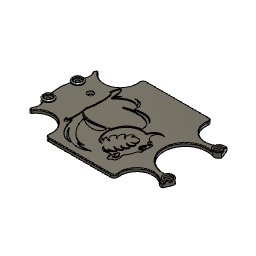
_chassis top.694dd02e-d549-4da8-af4c-a41191be3cab (Autodesk Fusion 360 design; units mm, degrees)
Autodesk Fusion 360 part; units mm, degrees
sketch "reference" plane through (0, 0, 0) normal (0, 1, 0) x (1, 0, 0)
  line L0 (26.708, 42.6236) -> (27.1586, 42.6236)
  line L1 (-27.225, -55.0823) -> (17.225, -55.0823)
  line L2 (17.225, -55.0823) -> (17.225, -42.3823)
  line L3 (17.225, -42.3823) -> (-27.225, -42.3823)
  line L4 (-27.225, -42.3823) -> (-27.225, -55.0823)
  circle A0 centre (0, 0) radius 65
  line L5 (-27.225, 55.0823) -> (17.225, 55.0823)
  line L6 (17.225, 55.0823) -> (17.225, 42.3823)
  line L7 (17.225, 42.3823) -> (-27.225, 42.3823)
  line L8 (-27.225, 55.0823) -> (-27.225, 42.3823)
  circle A1 centre (0, 0) radius 67.15
  circle A2 centre (68.0978, 18.2467) radius 3
  circle A3 centre (68.0978, 18.2467) radius 1.425
  line L9 (0, 0) -> (82, 0) construction
  line L10 (0, 0) -> (-41, 71.0141) construction
  line L11 (0, 0) -> (-41, -71.0141) construction
  line L12 (87.4769, -0.0257) -> (79.614, 0.0081)
  line L13 (-39.814, 68.9437) -> (-43.7162, 75.77)
  line L14 (-39.8, -68.9518) -> (-43.7607, -75.7444)
  line L15 (0, 0) -> (70.5, 0) construction
  arc A4 (79.614, 0.0081) -> (74.6944, -3.9877) centre (79.5926, -4.9919) ccw
  arc A5 (-39.814, 68.9437) -> (-33.8938, 66.6811) centre (-35.4732, 71.4251) ccw
  arc A6 (-39.8, -68.9518) -> (-40.8007, -62.6934) centre (-44.1194, -66.4332) ccw
  spline S0 degree 5 poles (-33.8938, 66.6811) (-33.483, 66.8179) (-33.0729, 66.9532) (-32.6634, 67.087) (-32.2547, 67.2193) (-31.8466, 67.3502) knots 0.021144 0.021144 0.021144 0.021144 0.021144 0.021144 0.032444 0.032444 0.032444 0.032444 0.032444 0.032444
  line L16 (-32.0549, 67.2834) -> (-31.6382, 67.417)
  spline S1 degree 5 poles (5.0849, 74.3263) (6.6179, 74.3731) (11.2429, 74.4207) (18.7539, 74.0099) (28.746, 72.2391) (40.5731, 67.6689) (52.3904, 59.5578) (62.916, 48.5693) (72.252, 34.9305) (78.8493, 22.0782) (83.3385, 11.4171) (86.1309, 3.8631) (87.4769, -0.0257) knots 0.251095 0.251095 0.251095 0.251095 0.251095 0.251095 0.3 0.4 0.5 0.6 0.7 0.8 0.9 1 1 1 1 1 1
  line L17 (-9.3123, 73.8863) -> (19.482, 74.7663)
  spline S2 degree 5 poles (-40.8007, -62.6934) (-41.1245, -62.4061) (-41.4467, -62.1186) (-41.7673, -61.8309) (-42.0863, -61.543) (-42.4037, -61.255) knots 0.021144 0.021144 0.021144 0.021144 0.021144 0.021144 0.032444 0.032444 0.032444 0.032444 0.032444 0.032444
  line L18 (-42.2416, -61.4021) -> (-42.5658, -61.1079)
  spline S3 degree 5 poles (-66.9109, -32.7595) (-67.718, -31.4553) (-70.0717, -27.4737) (-73.4714, -20.7636) (-76.9339, -11.2248) (-78.8895, 1.3029) (-77.7737, 15.5925) (-73.5202, 30.2022) (-66.3767, 45.1068) (-58.5449, 57.2464) (-51.5568, 66.4647) (-46.4109, 72.66) (-43.7162, 75.77) knots 0.251095 0.251095 0.251095 0.251095 0.251095 0.251095 0.3 0.4 0.5 0.6 0.7 0.8 0.9 1 1 1 1 1 1
  line L19 (-59.9171, -44.0611) -> (-73.9047, -21.4578)
  arc A7 (-66.9109, -32.7595) -> (-37.25, -64.5189) centre (0, 0) ccw
  spline S4 degree 5 poles (74.6944, -3.9877) (74.6075, -4.4118) (74.5196, -4.8346) (74.4308, -5.2561) (74.341, -5.6763) (74.2503, -6.0951) knots 0.021144 0.021144 0.021144 0.021144 0.021144 0.021144 0.032444 0.032444 0.032444 0.032444 0.032444 0.032444
  line L20 (74.2965, -5.8814) -> (74.204, -6.3089)
  spline S5 degree 5 poles (61.826, -41.5668) (61.1001, -42.9178) (58.8287, -46.947) (54.7175, -53.2463) (48.1879, -61.0143) (38.3164, -68.9717) (25.3834, -75.1503) (10.6042, -78.7715) (-5.8753, -80.0373) (-20.3044, -79.3246) (-31.7817, -77.8819) (-39.7199, -76.523) (-43.7607, -75.7444) knots 0.251095 0.251095 0.251095 0.251095 0.251095 0.251095 0.3 0.4 0.5 0.6 0.7 0.8 0.9 1 1 1 1 1 1
  line L21 (68.2252, -29.657) -> (55.4268, -53.4766)
  arc A8 (61.826, -41.5668) -> (74.5, 0) centre (0, 0) ccw
  arc A9 (5.0849, 74.3263) -> (-37.25, 64.5189) centre (0, 0) ccw
  circle A10 centre (18.2467, 68.0978) radius 3
  circle A11 centre (18.2467, 68.0978) radius 1.425
  circle A12 centre (-49.851, 49.851) radius 3
  circle A13 centre (-49.851, 49.851) radius 1.425
  circle A14 centre (-68.0978, -18.2467) radius 3
  circle A15 centre (-68.0978, -18.2467) radius 1.425
  circle A16 centre (-18.2467, -68.0978) radius 3
  circle A17 centre (-18.2467, -68.0978) radius 1.425
  circle A18 centre (49.851, -49.851) radius 3
  circle A19 centre (49.851, -49.851) radius 1.425
  line L22 (0, 0) -> (55.15, 0) construction
  line L23 (0, 0) -> (55.15, 0) construction
  circle A20 centre (42.2474, -35.4497) radius 12
  circle A21 centre (42.2474, 35.4497) radius 12
  line L24 (0, 0) -> (55.15, 0) construction
  line L25 (0, 0) -> (55.15, 0) construction
  circle A22 centre (-42.2474, 35.4497) radius 12
  circle A23 centre (-42.2474, -35.4497) radius 12
  circle A24 centre (0, 0) radius 62.5
  line L26 (-5, -42.3823) -> (-5, 42.3823)
  point P0 (39, 67.55)
  point P1 (-78, 0)
  point P2 (39, -67.55)
  dimension "d9" = 12.7
  dimension "d10" = 44.45
  dimension "d53" = 12.7
  dimension "d54" = 44.45
  dimension "d63" = 130
  dimension "d76" = 134.3
  dimension "d123" = 78
  dimension "d127" = 5
  dimension "d128" = 5
  dimension "d129" = 5
  dimension "d132" = 149
  dimension "d136" = 360
  dimension "d204" = 55.15
  dimension "d206" = 55.15
  dimension "d207" = 24
  dimension "d208" = 24
  dimension "d210" = 55.15
  dimension "d212" = 55.15
  dimension "d213" = 24
  dimension "d214" = 24
  dimension "d227" = 125
  dimension "d232" = 84.7646
  constraint perpendicular L1 L2
  constraint perpendicular L2 L3
  constraint coincident A0.centre A1.centre
  constraint perpendicular L5 L6
  constraint perpendicular L6 L7
  constraint horizontal L9
  constraint horizontal L15
  constraint tangent A4 S4
  constraint tangent L12 A4
  constraint tangent A5 S0
  constraint tangent L13 A5
  constraint tangent A6 S2
  constraint tangent L14 A6
  constraint coincident S0.end A7
  constraint midpoint S0.end L16
  constraint coincident S1.start A7
  constraint midpoint S1.start L17
  constraint coincident L10 A9.end
  constraint coincident S2.end A7
  constraint midpoint S2.end L18
  constraint midpoint S3.start L19
  constraint coincident L11 A7.end
  constraint concentric A7 A8
  constraint coincident S4.end A8
  constraint midpoint S4.end L20
  constraint midpoint S5.start L21
  constraint coincident L9 A8.end
  constraint concentric A8 A9
  constraint horizontal L22
  constraint horizontal L23
  constraint horizontal L24
  constraint horizontal L25
  constraint midpoint L3 L26.start
  constraint midpoint L7 L26.end
  constraint perpendicular L7 L26
  measures "d9" distance of L1.end L2.end
  measures "d10" distance of L2.end L3.end
  measures "d53" distance of L5.end L6.end
  measures "d54" distance of L6.end L7.end
  measures "d63" diameter of A0
  measures "d76" diameter of A1
  measures "d123" distance of A0.centre P0
  measures "d127" radius of A4
  measures "d128" radius of A5
  measures "d129" radius of A6
  measures "d132" diameter of A7
  measures "d204" distance of A0.centre A20.centre
  measures "d206" distance of A0.centre A21.centre
  measures "d207" diameter of A20
  measures "d208" diameter of A21
  measures "d210" distance of A0.centre A23.centre
  measures "d212" distance of A0.centre A22.centre
  measures "d213" diameter of A22
  measures "d214" diameter of A23
  measures "d227" diameter of A24
  measures "d232" distance of L26.start L26.end
sketch "Sketch6" plane through (0, 0, 0) normal (0, 1, 0) x (1, 0, 0)
  line L0 (25.9471, -41.0033) -> (-25.9305, -41.0033)
  arc A0 (53.3928, 17.0259) -> (53.3489, -17.1529) centre (47.6253, -0.0562) ccw
  arc A1 (-28.8946, -37.5404) -> (-53.2717, -27.6825) centre (-42.2338, -35.4569) ccw
  arc A2 (52.1423, -26.2602) -> (28.9106, -37.5367) centre (42.2443, -35.4374) ccw
  arc A3 (55.1761, 27.1684) -> (52.1143, 26.331) centre (54.3168, 24.2941) ccw
  arc A4 (52.1423, -26.2602) -> (55.2056, -27.0935) centre (54.3422, -24.2205) ccw
  arc A5 (58.3345, -19.4651) -> (53.3489, -17.1529) centre (54.6188, -20.946) ccw
  arc A6 (53.3928, 17.0259) -> (58.3852, 19.3275) centre (54.6724, 20.8157) ccw
  circle A7 centre (54.6724, 20.8157) radius 1.425
  circle A8 centre (54.6188, -20.946) radius 1.425
  arc A9 (-56.1762, -2.0025) -> (-56.1762, -2.0026) centre (-0.0106, -0.0004) ccw
  circle A10 centre (-54.8812, 12.3936) radius 1.425
  circle A11 centre (-54.8757, -12.1807) radius 1.425
  arc A12 (28.9662, 37.5373) -> (52.1143, 26.331) centre (42.246, 35.4576) ccw
  line L1 (-54.6751, -2.0026) -> (-54.4366, -2.0026) construction
  line L2 (-49.9389, 12.059) -> (-49.9913, 12.0592)
  line L3 (-44.9427, 8.8286) -> (-44.9427, 8.8286)
  spline S0 degree 5 poles (-38.2674, -23.601) (-38.2616, -23.5615) (-38.25, -23.4822) (-38.2328, -23.3629) (-38.21, -23.2029) (-38.1818, -23.0019) (-38.1594, -22.8402) (-38.1427, -22.7184) (-38.1316, -22.6368) (-38.1261, -22.596) knots 0 0 0 0 0 0 0.2 0.4 0.6 0.8 1 1 1 1 1 1
  line L4 (-38.2822, -23.7022) -> (-38.2526, -23.4999)
  line L5 (-38.1402, -22.7004) -> (-38.112, -22.4916)
  arc A13 (-53.2884, 27.6676) -> (-28.8973, 37.5386) centre (-42.2488, 35.4595) ccw
  line L6 (-54.333, 19.0252) -> (-54.7513, 17.7702)
  arc A14 (-56.8345, 14.6706) -> (-57.7304, 11.4541) centre (-54.8812, 12.3936) ccw
  spline S1 degree 3 poles (-57.5488, 7.7264) (-57.7948, 6.6323) (-57.9976, 5.5893) (-58.1533, 4.5869) (-58.73, 0.873) (-58.6151, -2.3643) (-57.8493, -6.2568) (-57.7624, -6.6981) (-57.6677, -7.149) (-57.5653, -7.6097) knots 0.254144 0.254144 0.254144 0.254144 0.280571 0.280571 0.280571 0.378481 0.378481 0.378481 0.389582 0.389582 0.389582 0.389582
  arc A15 (-57.7325, -11.2651) -> (-56.8532, -14.4367) centre (-54.8757, -12.1807) ccw
  spline S2 degree 3 poles (-54.8028, -17.5596) (-54.6442, -18.0533) (-54.4816, -18.5512) (-54.3154, -19.0517) knots 0.459488 0.459488 0.459488 0.459488 0.468931 0.468931 0.468931 0.468931
  arc A16 (-55.114, 16.8875) -> (-54.7513, 17.7702) centre (-61.3921, 19.9836) ccw
  arc A17 (-54.333, 19.0252) -> (-55.3983, 25.4709) centre (-60.9739, 21.2385) ccw
  arc A18 (-57.5488, 7.7264) -> (-57.4036, 8.667) centre (-64.3783, 9.2621) ccw
  arc A19 (-57.4291, -8.4753) -> (-57.5653, -7.6097) centre (-64.3985, -9.1286) ccw
  arc A20 (-54.8028, -17.5596) -> (-55.1565, -16.672) centre (-61.4673, -19.7007) ccw
  arc A21 (-55.3823, -25.4886) -> (-54.3154, -19.0517) centre (-60.9588, -21.2575) ccw
  arc A22 (-51.9311, -12.9587) -> (-51.9223, -12.9246) centre (-54.8757, -12.1807) ccw
  line L7 (-53.5111, 9.0025) -> (-53.3775, 9.0028)
  arc A23 (-53.5111, 9.0025) -> (-54.0242, 8.7111) centre (-53.5096, 8.4025) ccw
  line L8 (-25.9331, 41.0003) -> (26.0023, 41.0015)
  arc A24 (-55.4878, -26.5244) -> (-54.9832, -27.5548) centre (-0.0035, 0.0074) ccw
  arc A25 (-54.9996, 27.5386) -> (-55.5043, 26.5064) centre (-0.0035, 0.0074) ccw
  arc A26 (-53.2884, 27.6676) -> (-54.9996, 27.5386) centre (-54.1054, 27.0909) ccw
  arc A27 (-55.5043, 26.5064) -> (-55.3983, 25.4709) centre (-54.6018, 26.0756) ccw
  arc A28 (-54.9832, -27.5548) -> (-53.2717, -27.6825) centre (-54.0893, -27.1066) ccw
  arc A29 (-55.3823, -25.4886) -> (-55.4878, -26.5244) centre (-54.5856, -26.093) ccw
  arc A30 (55.2056, -27.0935) -> (58.3345, -19.4651) centre (-0.0035, 0.0074) ccw
  arc A31 (58.3852, 19.3275) -> (55.1761, 27.1684) centre (-0.0035, 0.0074) ccw
  arc A32 (-28.8946, -37.5404) -> (-25.9305, -41.0033) centre (-25.9305, -38.0033) ccw
  arc A33 (25.9471, -41.0033) -> (28.9106, -37.5367) centre (25.9471, -38.0033) ccw
  arc A34 (28.9662, 37.5373) -> (26.0023, 41.0015) centre (26.0024, 38.0015) ccw
  arc A35 (-25.9331, 41.0003) -> (-28.8973, 37.5386) centre (-25.9331, 38.0003) ccw
  circle A36 centre (-54.8812, 12.3936) radius 3
  circle A37 centre (-54.8757, -12.1807) radius 3
  circle A38 centre (-54.8812, 12.3936) radius 4.5
  circle A39 centre (-54.8757, -12.1807) radius 4.5
  arc A40 (51.5521, -17.6527) -> (56.0971, -25.1962) centre (54.6188, -20.946) ccw
  arc A41 (56.1643, 25.0612) -> (51.5973, 17.5303) centre (54.6724, 20.8157) ccw
  arc A42 (57.2747, 22.4063) -> (57.6738, 21.3577) centre (54.6724, 20.8157) ccw
  arc A43 (57.6206, -21.4861) -> (57.2117, -22.552) centre (54.6188, -20.946) ccw
  circle A44 centre (-40.8812, 8.8936) radius 2.5
  spline S3 degree 3 poles (23.3331, -3.4893) (23.2569, -3.2607) (23.0664, -2.9273) (22.895, -2.7559) knots 0 0 0 0 1 1 1 1
  spline S4 degree 3 poles (22.895, -2.7559) (22.1997, -2.0415) (21.2948, -2.2891) (20.3042, -3.4798) knots 0 0 0 0 1 1 1 1
  line L9 (20.3042, -3.4798) -> (20.0375, -3.7941)
  line L10 (20.0375, -3.7941) -> (19.7803, -3.556)
  spline S5 degree 3 poles (19.7803, -3.556) (19.6374, -3.4321) (19.4088, -3.2512) (19.2755, -3.1654) knots 0 0 0 0 1 1 1 1
  spline S6 degree 3 poles (19.2755, -3.1654) (19.0374, -3.0226) (18.5516, -2.3653) (18.6278, -2.2987) knots 0 0 0 0 1 1 1 1
  spline S7 degree 3 poles (18.6278, -2.2987) (18.6468, -2.2891) (18.8564, -2.1748) (19.0945, -2.0605) knots 0 0 0 0 1 1 1 1
  spline S8 degree 3 poles (19.0945, -2.0605) (19.5708, -1.8224) (20.7138, -1.0795) (20.7138, -1.0033) knots 0 0 0 0 1 1 1 1
  spline S9 degree 3 poles (20.7138, -1.0033) (20.7138, -0.9747) (20.5137, -0.9652) (20.2661, -0.9842) knots 0 0 0 0 1 1 1 1
  spline S10 degree 3 poles (20.2661, -0.9842) (19.647, -1.0318) (18.6087, -0.7747) (17.942, -0.4222) knots 0 0 0 0 1 1 1 1
  spline S11 degree 3 poles (17.942, -0.4222) (16.9228, 0.1302) (16.0179, 1.2923) (15.7036, 2.4734) knots 0 0 0 0 1 1 1 1
  spline S12 degree 3 poles (15.7036, 2.4734) (15.5322, 3.1115) (15.5417, 4.1593) (15.7131, 4.8546) knots 0 0 0 0 1 1 1 1
  spline S13 degree 3 poles (15.7131, 4.8546) (16.1703, 6.6072) (17.6753, 8.0074) (19.5136, 8.3979) knots 0 0 0 0 1 1 1 1
  spline S14 degree 3 poles (19.5136, 8.3979) (19.9137, 8.4836) (20.3994, 8.5122) (20.7138, 8.4836) knots 0 0 0 0 1 1 1 1
  line L11 (20.7138, 8.4836) -> (21.2376, 8.4265)
  line L12 (21.2376, 8.4265) -> (20.8852, 8.617)
  spline S15 degree 3 poles (20.8852, 8.617) (19.7803, 9.2075) (17.9134, 9.2552) (16.5609, 8.7218) knots 0 0 0 0 1 1 1 1
  spline S16 degree 3 poles (16.5609, 8.7218) (14.694, 7.9979) (13.2747, 6.6644) (12.3889, 4.8165) knots 0 0 0 0 1 1 1 1
  spline S17 degree 3 poles (12.3889, 4.8165) (12.2079, 4.426) (12.0079, 3.8926) (11.9412, 3.6164) knots 0 0 0 0 1 1 1 1
  line L13 (11.9412, 3.6164) -> (11.8269, 3.1115)
  line L14 (11.8269, 3.1115) -> (11.2935, 3.2925)
  spline S18 degree 3 poles (11.2935, 3.2925) (9.579, 3.8831) (6.9692, 4.0736) (5.1309, 3.7307) knots 0 0 0 0 1 1 1 1
  spline S19 degree 3 poles (5.1309, 3.7307) (-2.8225, 2.2638) (-8.0613, -6.3468) (-6.2229, -14.9098) knots 0 0 0 0 1 1 1 1
  spline S20 degree 3 poles (-6.2229, -14.9098) (-5.8801, -16.5195) (-5.1943, -18.3673) (-4.2322, -20.32) knots 0 0 0 0 1 1 1 1
  spline S21 degree 3 poles (-4.2322, -20.32) (-3.6226, -21.5392) (-2.4034, -22.4345) (-1.2318, -22.5107) knots 0 0 0 0 1 1 1 1
  spline S22 degree 3 poles (-1.2318, -22.5107) (-0.6318, -22.5488) (-0.0508, -22.425) (0.1207, -22.2154) knots 0 0 0 0 1 1 1 1
  spline S23 degree 3 poles (0.1207, -22.2154) (0.1969, -22.1297) (0.1112, -22.1011) (-0.1841, -22.0916) knots 0 0 0 0 1 1 1 1
  spline S24 degree 3 poles (-0.1841, -22.0916) (-1.6891, -22.0535) (-3.1845, -20.4724) (-3.4131, -18.7007) knots 0 0 0 0 1 1 1 1
  spline S25 degree 3 poles (-3.4131, -18.7007) (-3.4512, -18.4245) (-3.4416, -18.2435) (-3.3845, -18.2435) knots 0 0 0 0 1 1 1 1
  spline S26 degree 3 poles (-3.3845, -18.2435) (-3.3274, -18.2435) (-3.2893, -18.3007) (-3.2893, -18.3769) knots 0 0 0 0 1 1 1 1
  spline S27 degree 3 poles (-3.2893, -18.3769) (-3.2893, -18.4531) (-3.0702, -18.7483) (-2.813, -19.0436) knots 0 0 0 0 1 1 1 1
  spline S28 degree 3 poles (-2.813, -19.0436) (-2.3368, -19.558) (-1.9176, -19.7866) (-1.2128, -19.9009) knots 0 0 0 0 1 1 1 1
  spline S29 degree 3 poles (-1.2128, -19.9009) (-0.8889, -19.958) (-0.7842, -19.8151) (-1.089, -19.7199) knots 0 0 0 0 1 1 1 1
  spline S30 degree 3 poles (-1.089, -19.7199) (-1.3747, -19.6342) (-2.0415, -18.8531) (-2.2415, -18.3864) knots 0 0 0 0 1 1 1 1
  spline S31 degree 3 poles (-2.2415, -18.3864) (-2.5082, -17.7768) (-2.6416, -16.8719) (-2.5653, -16.2814) knots 0 0 0 0 1 1 1 1
  line L15 (-2.5654, -16.2814) -> (-2.5082, -15.7575)
  line L16 (-2.5082, -15.7575) -> (-2.1843, -16.1385)
  spline S32 degree 3 poles (-2.1843, -16.1385) (-1.4033, -17.0529) (-0.0222, -17.672) (1.2256, -17.672) knots 0 0 0 0 1 1 1 1
  spline S33 degree 3 poles (1.2256, -17.672) (2.0162, -17.672) (2.3496, -17.5387) (1.7876, -17.4529) knots 0 0 0 0 1 1 1 1
  spline S34 degree 3 poles (1.7876, -17.4529) (0.8256, -17.3005) (-0.4984, -16.2718) (-0.9937, -15.3098) knots 0 0 0 0 1 1 1 1
  spline S35 degree 3 poles (-0.9937, -15.3098) (-1.8986, -13.5477) (-1.4033, -11.6427) (0.1588, -10.8712) knots 0 0 0 0 1 1 1 1
  line L17 (0.1588, -10.8712) -> (0.6446, -10.6235)
  line L18 (0.6446, -10.6235) -> (0.9494, -11.0807)
  spline S36 degree 3 poles (0.9494, -11.0807) (1.359, -11.6808) (2.0162, -12.2713) (2.6067, -12.5666) knots 0 0 0 0 1 1 1 1
  spline S37 degree 3 poles (2.6067, -12.5666) (2.8734, -12.7) (3.1116, -12.8143) (3.1497, -12.8143) knots 0 0 0 0 1 1 1 1
  spline S38 degree 3 poles (3.1497, -12.8143) (3.1878, -12.8143) (3.0163, -12.6047) (2.7782, -12.3475) knots 0 0 0 0 1 1 1 1
  spline S39 degree 3 poles (2.7782, -12.3475) (1.178, -10.6426) (1.3209, -7.8898) (3.083, -6.5563) knots 0 0 0 0 1 1 1 1
  spline S40 degree 3 poles (3.083, -6.5563) (3.3021, -6.3849) (3.5402, -6.242) (3.6164, -6.242) knots 0 0 0 0 1 1 1 1
  spline S41 degree 3 poles (3.6164, -6.242) (3.6831, -6.242) (3.7878, -6.442) (3.845, -6.6802) knots 0 0 0 0 1 1 1 1
  spline S42 degree 3 poles (3.845, -6.6802) (4.1879, -8.0422) (5.4357, -9.3472) (6.6644, -9.6329) knots 0 0 0 0 1 1 1 1
  spline S43 degree 3 poles (6.6644, -9.6329) (6.9501, -9.6996) (6.9501, -9.6901) (6.5501, -9.3472) knots 0 0 0 0 1 1 1 1
  spline S44 degree 3 poles (6.5501, -9.3472) (5.3118, -8.2708) (4.8546, -6.3849) (5.4928, -4.9942) knots 0 0 0 0 1 1 1 1
  spline S45 degree 3 poles (5.4928, -4.9942) (6.0072, -3.8798) (6.7501, -3.3845) (7.9122, -3.3845) knots 0 0 0 0 1 1 1 1
  spline S46 degree 3 poles (7.9122, -3.3845) (8.2932, -3.3845) (8.6361, -3.4321) (8.6646, -3.4798) knots 0 0 0 0 1 1 1 1
  spline S47 degree 3 poles (8.6646, -3.4798) (8.6932, -3.5369) (8.6361, -3.7084) (8.5218, -3.8608) knots 0 0 0 0 1 1 1 1
  spline S48 degree 3 poles (8.5218, -3.8608) (8.2646, -4.2227) (7.9503, -5.1085) (7.9503, -5.4514) knots 0 0 0 0 1 1 1 1
  spline S49 degree 3 poles (7.9503, -5.4514) (7.9598, -5.7181) (7.9598, -5.7181) (8.1408, -5.3752) knots 0 0 0 0 1 1 1 1
  spline S50 degree 3 poles (8.1408, -5.3752) (8.5408, -4.6228) (9.5695, -3.956) (10.6649, -3.756) knots 0 0 0 0 1 1 1 1
  spline S51 degree 3 poles (10.6649, -3.756) (11.7126, -3.5655) (12.989, -3.9465) (13.7224, -4.6799) knots 0 0 0 0 1 1 1 1
  spline S52 degree 3 poles (13.7224, -4.6799) (15.2369, -6.2039) (14.4939, -8.6423) (12.2841, -9.3853) knots 0 0 0 0 1 1 1 1
  line L19 (12.2841, -9.3853) -> (11.7126, -9.5758)
  line L20 (11.7126, -9.5758) -> (12.4746, -9.5472)
  spline S53 degree 3 poles (12.4746, -9.5472) (13.2938, -9.4996) (14.0653, -9.2614) (14.6749, -8.8519) knots 0 0 0 0 1 1 1 1
  spline S54 degree 3 poles (14.6749, -8.8519) (15.0845, -8.5756) (15.1321, -8.6137) (15.275, -9.29) knots 0 0 0 0 1 1 1 1
  spline S55 degree 3 poles (15.275, -9.29) (15.456, -10.1187) (15.0369, -11.1474) (14.3034, -11.6808) knots 0 0 0 0 1 1 1 1
  spline S56 degree 3 poles (14.3034, -11.6808) (13.1985, -12.4809) (11.7984, -12.6142) (10.5982, -12.0142) knots 0 0 0 0 1 1 1 1
  spline S57 degree 3 poles (10.5982, -12.0142) (10.341, -11.8999) (10.141, -11.8237) (10.141, -11.8713) knots 0 0 0 0 1 1 1 1
  spline S58 degree 3 poles (10.141, -11.8713) (10.141, -12.0618) (11.2459, -12.919) (11.7412, -13.1095) knots 0 0 0 0 1 1 1 1
  spline S59 degree 3 poles (11.7412, -13.1095) (12.3794, -13.3477) (13.4462, -13.4429) (14.0463, -13.3) knots 0 0 0 0 1 1 1 1
  spline S60 degree 3 poles (14.0463, -13.3) (14.2749, -13.2524) (14.4844, -13.2238) (14.5035, -13.2334) knots 0 0 0 0 1 1 1 1
  spline S61 degree 3 poles (14.5035, -13.2334) (14.6273, -13.3572) (14.6178, -14.0239) (14.4749, -14.4811) knots 0 0 0 0 1 1 1 1
  spline S62 degree 3 poles (14.4749, -14.4811) (13.9796, -16.1956) (11.5126, -17.0529) (9.7886, -16.1004) knots 0 0 0 0 1 1 1 1
  spline S63 degree 3 poles (9.7886, -16.1004) (9.56, -15.9766) (9.379, -15.9099) (9.379, -15.948) knots 0 0 0 0 1 1 1 1
  spline S64 degree 3 poles (9.379, -15.948) (9.379, -16.129) (10.3791, -16.9386) (10.884, -17.1767) knots 0 0 0 0 1 1 1 1
  spline S65 degree 3 poles (10.884, -17.1767) (11.3697, -17.4053) (11.5412, -17.4339) (12.4461, -17.4339) knots 0 0 0 0 1 1 1 1
  spline S66 degree 3 poles (12.4461, -17.4339) (13.2081, -17.4339) (13.4748, -17.4625) (13.4748, -17.5577) knots 0 0 0 0 1 1 1 1
  spline S67 degree 3 poles (13.4748, -17.5577) (13.4748, -17.8339) (13.0176, -18.615) (12.608, -19.0246) knots 0 0 0 0 1 1 1 1
  spline S68 degree 3 poles (12.608, -19.0246) (11.4078, -20.2247) (9.4742, -20.4914) (7.8264, -19.6723) knots 0 0 0 0 1 1 1 1
  line L21 (7.8264, -19.6723) -> (7.2835, -19.396)
  line L22 (7.2835, -19.396) -> (7.474, -19.6723)
  spline S69 degree 3 poles (7.474, -19.6723) (8.1693, -20.6438) (9.56, -21.3201) (10.9221, -21.3296) knots 0 0 0 0 1 1 1 1
  spline S70 degree 3 poles (10.9221, -21.3296) (11.3316, -21.3391) (11.665, -21.3487) (11.665, -21.3677) knots 0 0 0 0 1 1 1 1
  spline S71 degree 3 poles (11.665, -21.3677) (11.665, -21.5392) (11.1602, -22.2821) (10.7697, -22.6726) knots 0 0 0 0 1 1 1 1
  spline S72 degree 3 poles (10.7697, -22.6726) (9.8743, -23.5775) (8.5884, -23.9966) (7.2359, -23.8537) knots 0 0 0 0 1 1 1 1
  spline S73 degree 3 poles (7.2359, -23.8537) (6.9216, -23.8156) (6.6549, -23.7966) (6.6358, -23.8156) knots 0 0 0 0 1 1 1 1
  spline S74 degree 3 poles (6.6358, -23.8156) (6.531, -23.9204) (8.0836, -24.5491) (8.5503, -24.5967) knots 0 0 0 0 1 1 1 1
  spline S75 degree 3 poles (8.5503, -24.5967) (9.0837, -24.6538) (9.0932, -24.6538) (8.9313, -24.8348) knots 0 0 0 0 1 1 1 1
  spline S76 degree 3 poles (8.9313, -24.8348) (8.8456, -24.9301) (8.5027, -25.1491) (8.1693, -25.3111) knots 0 0 0 0 1 1 1 1
  spline S77 degree 3 poles (8.1693, -25.3111) (6.5977, -26.0826) (4.5403, -25.6063) (3.2925, -24.1871) knots 0 0 0 0 1 1 1 1
  spline S78 degree 3 poles (3.2925, -24.1871) (2.8258, -23.6537) (2.8258, -23.7871) (3.283, -24.7681) knots 0 0 0 0 1 1 1 1
  spline S79 degree 3 poles (3.283, -24.7681) (3.7878, -25.8635) (4.826, -26.7398) (6.0643, -27.1113) knots 0 0 0 0 1 1 1 1
  spline S80 degree 3 poles (6.0643, -27.1113) (7.0644, -27.4161) (8.3312, -27.3494) (9.2361, -26.9303) knots 0 0 0 0 1 1 1 1
  spline S81 degree 3 poles (9.2361, -26.9303) (9.6076, -26.7589) (10.2267, -26.5398) (10.6173, -26.435) knots 0 0 0 0 1 1 1 1
  spline S82 degree 3 poles (10.6173, -26.435) (11.0078, -26.3398) (11.4174, -26.2255) (11.5221, -26.1969) knots 0 0 0 0 1 1 1 1
  spline S83 degree 3 poles (11.5221, -26.1969) (11.7031, -26.1397) (11.7126, -26.1969) (11.7412, -26.9779) knots 0 0 0 0 1 1 1 1
  spline S84 degree 3 poles (11.7412, -26.9779) (11.8174, -28.921) (12.4461, -30.5784) (13.3128, -31.1023) knots 0 0 0 0 1 1 1 1
  spline S85 degree 3 poles (13.3128, -31.1023) (13.6748, -31.3309) (14.3225, -31.3499) (14.7035, -31.1499) knots 0 0 0 0 1 1 1 1
  spline S86 degree 3 poles (14.7035, -31.1499) (15.0464, -30.9784) (15.6083, -30.3212) (15.837, -29.8545) knots 0 0 0 0 1 1 1 1
  spline S87 degree 3 poles (15.837, -29.8545) (15.9989, -29.5021) (15.9989, -29.5021) (16.4847, -29.5497) knots 0 0 0 0 1 1 1 1
  spline S88 degree 3 poles (16.4847, -29.5497) (17.3229, -29.6354) (17.761, -29.2544) (18.0849, -28.159) knots 0 0 0 0 1 1 1 1
  spline S89 degree 3 poles (18.0849, -28.159) (18.4659, -26.8636) (18.3325, -25.0729) (17.7134, -23.2251) knots 0 0 0 0 1 1 1 1
  line L23 (17.7134, -23.2251) -> (17.38, -22.225)
  line L24 (17.38, -22.225) -> (17.7515, -21.7773)
  spline S90 degree 3 poles (17.7515, -21.7773) (18.8183, -20.5009) (19.8946, -18.5293) (20.4661, -16.8148) knots 0 0 0 0 1 1 1 1
  spline S91 degree 3 poles (20.4661, -16.8148) (20.7995, -15.8146) (21.19, -14.1001) (21.19, -13.6334) knots 0 0 0 0 1 1 1 1
  spline S92 degree 3 poles (21.19, -13.6334) (21.19, -13.3953) (21.2186, -13.3858) (21.6663, -13.3858) knots 0 0 0 0 1 1 1 1
  spline S93 degree 3 poles (21.6663, -13.3858) (22.3235, -13.3858) (22.6473, -13.1953) (22.914, -12.6523) knots 0 0 0 0 1 1 1 1
  spline S94 degree 3 poles (22.914, -12.6523) (23.1141, -12.2428) (23.1426, -12.0713) (23.1426, -11.0045) knots 0 0 0 0 1 1 1 1
  spline S95 degree 3 poles (23.1426, -11.0045) (23.1331, -10.0996) (23.0855, -9.6329) (22.9331, -9.0614) knots 0 0 0 0 1 1 1 1
  spline S96 degree 3 poles (22.9331, -9.0614) (22.7426, -8.3661) (22.7331, -8.2804) (22.8664, -8.0232) knots 0 0 0 0 1 1 1 1
  spline S97 degree 3 poles (22.8664, -8.0232) (22.9521, -7.8708) (23.1236, -7.3374) (23.2474, -6.8421) knots 0 0 0 0 1 1 1 1
  spline S98 degree 3 poles (23.2474, -6.8421) (23.5141, -5.7943) (23.5522, -4.1941) (23.3331, -3.4893) knots 0 0 0 0 1 1 1 1
  spline S99 degree 3 poles (23.0474, -6.9564) (22.7045, -8.2994) (21.6567, -9.8139) (20.6661, -10.3949) knots 0 0 0 0 1 1 1 1
  spline S100 degree 3 poles (20.6661, -10.3949) (20.1804, -10.6807) (19.5136, -10.7759) (19.1898, -10.6045) knots 0 0 0 0 1 1 1 1
  spline S101 degree 3 poles (19.1898, -10.6045) (18.5706, -10.2711) (18.3325, -9.4329) (18.5611, -8.328) knots 0 0 0 0 1 1 1 1
  spline S102 degree 3 poles (18.5611, -8.328) (18.9326, -6.5754) (20.3232, -4.7656) (21.5901, -4.4323) knots 0 0 0 0 1 1 1 1
  spline S103 degree 3 poles (21.5901, -4.4323) (22.8188, -4.0989) (23.4855, -5.2514) (23.0474, -6.9564) knots 0 0 0 0 1 1 1 1
  spline S104 degree 3 poles (15.8846, -26.2636) (15.6369, -26.6827) (15.1512, -26.7398) (14.7416, -26.3969) knots 0 0 0 0 1 1 1 1
  spline S105 degree 3 poles (14.7416, -26.3969) (14.1225, -25.8826) (13.5986, -24.3776) (13.7034, -23.4346) knots 0 0 0 0 1 1 1 1
  spline S106 degree 3 poles (13.7034, -23.4346) (13.7415, -23.0632) (13.7319, -22.9965) (13.6462, -23.1394) knots 0 0 0 0 1 1 1 1
  spline S107 degree 3 poles (13.6462, -23.1394) (13.5891, -23.2441) (13.5605, -23.6632) (13.5891, -24.1871) knots 0 0 0 0 1 1 1 1
  spline S108 degree 3 poles (13.5891, -24.1871) (13.6176, -24.911) (13.6748, -25.1587) (13.9129, -25.673) knots 0 0 0 0 1 1 1 1
  spline S109 degree 3 poles (13.9129, -25.673) (14.0748, -26.0159) (14.3511, -26.435) (14.532, -26.6065) knots 0 0 0 0 1 1 1 1
  line L25 (14.532, -26.6065) -> (14.8463, -26.9113)
  line L26 (14.8463, -26.9113) -> (14.5892, -27.1684)
  spline S110 degree 3 poles (14.5892, -27.1684) (14.3034, -27.4542) (13.7891, -27.5209) (13.5224, -27.2923) knots 0 0 0 0 1 1 1 1
  spline S111 degree 3 poles (13.5224, -27.2923) (13.0366, -26.8827) (12.7413, -25.6349) (12.9033, -24.6157) knots 0 0 0 0 1 1 1 1
  spline S112 degree 3 poles (12.9033, -24.6157) (13.0271, -23.7775) (13.2652, -23.2727) (13.8081, -22.7012) knots 0 0 0 0 1 1 1 1
  spline S113 degree 3 poles (13.8081, -22.7012) (14.3701, -22.0916) (14.6082, -22.0916) (15.1797, -22.7012) knots 0 0 0 0 1 1 1 1
  spline S114 degree 3 poles (15.1797, -22.7012) (15.5988, -23.1203) (15.9417, -23.8728) (16.0846, -24.6253) knots 0 0 0 0 1 1 1 1
  spline S115 degree 3 poles (16.0846, -24.6253) (16.1703, -25.092) (16.0656, -25.9588) (15.8846, -26.2636) knots 0 0 0 0 1 1 1 1
  spline S116 degree 3 poles (21.0567, -5.9848) (20.4471, -4.6609) (18.5516, -7.204) (18.7421, -9.0805) knots 0 0 0 0 1 1 1 1
  spline S117 degree 3 poles (18.7421, -9.0805) (18.9516, -11.0807) (21.009, -9.2614) (21.1519, -6.9564) knots 0 0 0 0 1 1 1 1
  spline S118 degree 3 poles (21.1519, -6.9564) (21.1805, -6.4992) (21.1519, -6.1944) (21.0567, -5.9848) knots 0 0 0 0 1 1 1 1
  spline S119 degree 3 poles (6.4834, 7.4454) (6.3024, 8.1788) (5.6547, 9.4457) (5.1213, 10.0934) knots 0 0 0 0 1 1 1 1
  spline S120 degree 3 poles (5.1213, 10.0934) (3.4545, 12.1317) (0.4731, 13.5033) (-3.3845, 14.0082) knots 0 0 0 0 1 1 1 1
  spline S121 degree 3 poles (-3.3845, 14.0082) (-4.9656, 14.2177) (-8.0327, 14.2177) (-9.8139, 14.0082) knots 0 0 0 0 1 1 1 1
  spline S122 degree 3 poles (-9.8139, 14.0082) (-12.1189, 13.7319) (-15.586, 12.9509) (-17.0529, 12.3699) knots 0 0 0 0 1 1 1 1
  spline S123 degree 3 poles (-17.0529, 12.3699) (-17.2624, 12.2937) (-17.3862, 12.2651) (-17.3291, 12.3318) knots 0 0 0 0 1 1 1 1
  spline S124 degree 3 poles (-17.3291, 12.3318) (-17.1577, 12.5032) (-14.2716, 13.7129) (-13.0048, 14.1415) knots 0 0 0 0 1 1 1 1
  spline S125 degree 3 poles (-13.0048, 14.1415) (-5.4609, 16.6752) (1.3971, 16.1227) (4.5498, 12.7127) knots 0 0 0 0 1 1 1 1
  spline S126 degree 3 poles (4.5498, 12.7127) (4.8451, 12.3889) (5.0928, 12.1603) (5.0928, 12.1984) knots 0 0 0 0 1 1 1 1
  spline S127 degree 3 poles (5.0928, 12.1984) (5.0928, 12.227) (4.9594, 12.5222) (4.788, 12.8461) knots 0 0 0 0 1 1 1 1
  spline S128 degree 3 poles (4.788, 12.8461) (4.5879, 13.2176) (4.1784, 13.7319) (3.6259, 14.2844) knots 0 0 0 0 1 1 1 1
  spline S129 degree 3 poles (3.6259, 14.2844) (2.6734, 15.2369) (1.7019, 15.8179) (0.3207, 16.2656) knots 0 0 0 0 1 1 1 1
  spline S130 degree 3 poles (0.3207, 16.2656) (-1.5081, 16.8657) (-4.4513, 17.0276) (-6.8611, 16.6752) knots 0 0 0 0 1 1 1 1
  spline S131 degree 3 poles (-6.8611, 16.6752) (-7.8612, 16.5228) (-10.2901, 15.9798) (-10.7283, 15.8084) knots 0 0 0 0 1 1 1 1
  spline S132 degree 3 poles (-10.7283, 15.8084) (-10.8711, 15.7512) (-10.8807, 15.7989) (-10.7949, 16.2084) knots 0 0 0 0 1 1 1 1
  spline S133 degree 3 poles (-10.7949, 16.2084) (-10.633, 16.98) (-10.6616, 18.9707) (-10.8426, 19.666) knots 0 0 0 0 1 1 1 1
  spline S134 degree 3 poles (-10.8426, 19.666) (-11.3855, 21.7615) (-12.7571, 23.1141) (-14.7383, 23.5332) knots 0 0 0 0 1 1 1 1
  spline S135 degree 3 poles (-14.7383, 23.5332) (-15.5098, 23.7046) (-17.4339, 23.6665) (-17.8625, 23.4855) knots 0 0 0 0 1 1 1 1
  spline S136 degree 3 poles (-17.8625, 23.4855) (-18.0911, 23.3808) (-18.0911, 23.3808) (-17.8149, 23.4284) knots 0 0 0 0 1 1 1 1
  spline S137 degree 3 poles (-17.8149, 23.4284) (-17.2815, 23.5236) (-16.1289, 23.295) (-15.4146, 22.9521) knots 0 0 0 0 1 1 1 1
  spline S138 degree 3 poles (-15.4146, 22.9521) (-14.062, 22.3235) (-12.9571, 20.8947) (-12.5856, 19.3326) knots 0 0 0 0 1 1 1 1
  spline S139 degree 3 poles (-12.5856, 19.3326) (-12.519, 19.0659) (-12.5285, 19.0659) (-13.0238, 19.5327) knots 0 0 0 0 1 1 1 1
  spline S140 degree 3 poles (-13.0238, 19.5327) (-13.6715, 20.1423) (-14.2049, 20.4566) (-15.1002, 20.7233) knots 0 0 0 0 1 1 1 1
  spline S141 degree 3 poles (-15.1002, 20.7233) (-16.0147, 20.9995) (-17.5387, 21.0186) (-18.7197, 20.7709) knots 0 0 0 0 1 1 1 1
  spline S142 degree 3 poles (-18.7197, 20.7709) (-21.7201, 20.1327) (-25.092, 18.0944) (-27.8257, 15.2655) knots 0 0 0 0 1 1 1 1
  line L27 (-27.8257, 15.2655) -> (-28.6924, 14.3701)
  line L28 (-28.6924, 14.3701) -> (-28.7972, 16.1037)
  spline S143 degree 3 poles (-28.7972, 16.1037) (-29.0163, 19.4946) (-29.3497, 21.5043) (-30.0164, 23.5713) knots 0 0 0 0 1 1 1 1
  spline S144 degree 3 poles (-30.0164, 23.5713) (-30.045, 23.6475) (-29.9974, 23.6094) (-29.9212, 23.476) knots 0 0 0 0 1 1 1 1
  spline S145 degree 3 poles (-29.9212, 23.476) (-29.3973, 22.6283) (-28.7877, 19.5708) (-28.5496, 16.5799) knots 0 0 0 0 1 1 1 1
  line L29 (-28.5496, 16.5799) -> (-28.4829, 15.7227)
  line L30 (-28.4829, 15.7227) -> (-27.8638, 16.5799)
  spline S146 degree 3 poles (-27.8638, 16.5799) (-27.1303, 17.5896) (-26.3493, 18.5135) (-25.5492, 19.3041) knots 0 0 0 0 1 1 1 1
  spline S147 degree 3 poles (-25.5492, 19.3041) (-25.1301, 19.7136) (-25.0539, 19.8184) (-25.292, 19.6565) knots 0 0 0 0 1 1 1 1
  spline S148 degree 3 poles (-25.292, 19.6565) (-25.473, 19.5327) (-26.1969, 18.8659) (-26.8827, 18.1706) knots 0 0 0 0 1 1 1 1
  spline S149 degree 3 poles (-26.8827, 18.1706) (-27.578, 17.4753) (-28.1495, 16.9419) (-28.1495, 16.98) knots 0 0 0 0 1 1 1 1
  spline S150 degree 3 poles (-28.1495, 16.98) (-28.1495, 17.1895) (-28.4543, 19.3326) (-28.5781, 20.047) knots 0 0 0 0 1 1 1 1
  spline S151 degree 3 poles (-28.5781, 20.047) (-28.902, 21.7901) (-29.5116, 23.476) (-29.9402, 23.7808) knots 0 0 0 0 1 1 1 1
  spline S152 degree 3 poles (-29.9402, 23.7808) (-30.045, 23.8475) (-30.1879, 24.038) (-30.2736, 24.1904) knots 0 0 0 0 1 1 1 1
  spline S153 degree 3 poles (-30.2736, 24.1904) (-30.5022, 24.6476) (-30.9118, 25) (-31.188, 25) knots 0 0 0 0 1 1 1 1
  spline S154 degree 3 poles (-31.188, 25) (-31.4833, 25) (-31.9404, 24.5714) (-32.1976, 24.0475) knots 0 0 0 0 1 1 1 1
  spline S155 degree 3 poles (-32.1976, 24.0475) (-32.6548, 23.1426) (-33.2263, 20.9805) (-33.4835, 19.1421) knots 0 0 0 0 1 1 1 1
  spline S156 degree 3 poles (-33.4835, 19.1421) (-33.5407, 18.723) (-33.6073, 18.2468) (-33.6454, 18.0944) knots 0 0 0 0 1 1 1 1
  line L31 (-33.6454, 18.0944) -> (-33.6931, 17.8086)
  line L32 (-33.6931, 17.8086) -> (-33.4168, 18.0658)
  spline S157 degree 3 poles (-33.4168, 18.0658) (-32.731, 18.7135) (-32.1405, 18.1515) (-31.6261, 16.3608) knots 0 0 0 0 1 1 1 1
  spline S158 degree 3 poles (-31.6261, 16.3608) (-30.3784, 12.0746) (-30.4736, 2.902) (-31.8166, -2.432) knots 0 0 0 0 1 1 1 1
  spline S159 degree 3 poles (-31.8166, -2.432) (-32.0357, -3.2892) (-32.0357, -3.3655) (-31.9024, -3.9846) knots 0 0 0 0 1 1 1 1
  spline S160 degree 3 poles (-31.9024, -3.9846) (-31.7119, -4.8895) (-31.3309, -7.8327) (-31.188, -9.4329) knots 0 0 0 0 1 1 1 1
  spline S161 degree 3 poles (-31.188, -9.4329) (-31.0356, -11.176) (-31.0356, -15.186) (-31.1785, -16.3385) knots 0 0 0 0 1 1 1 1
  spline S162 degree 3 poles (-31.1785, -16.3385) (-31.3404, -17.5768) (-31.6547, -18.6817) (-31.9309, -19.015) knots 0 0 0 0 1 1 1 1
  spline S163 degree 3 poles (-31.9309, -19.015) (-32.3691, -19.5294) (-32.893, -19.3103) (-33.3502, -18.415) knots 0 0 0 0 1 1 1 1
  spline S164 degree 3 poles (-33.3502, -18.415) (-33.4359, -18.2626) (-33.5121, -18.1483) (-33.5407, -18.1768) knots 0 0 0 0 1 1 1 1
  spline S165 degree 3 poles (-33.5407, -18.1768) (-33.6264, -18.2626) (-33.0073, -20.4724) (-32.712, -21.1105) knots 0 0 0 0 1 1 1 1
  spline S166 degree 3 poles (-32.712, -21.1105) (-31.8071, -23.0632) (-30.7498, -22.2154) (-29.9116, -18.8722) knots 0 0 0 0 1 1 1 1
  spline S167 degree 3 poles (-29.9116, -18.8722) (-29.7783, -18.3578) (-29.6735, -17.853) (-29.6735, -17.7577) knots 0 0 0 0 1 1 1 1
  spline S168 degree 3 poles (-29.6735, -17.7577) (-29.6735, -17.653) (-29.6449, -17.5768) (-29.5973, -17.5768) knots 0 0 0 0 1 1 1 1
  spline S169 degree 3 poles (-29.5973, -17.5768) (-29.5592, -17.5768) (-29.4354, -18.0721) (-29.3116, -18.6817) knots 0 0 0 0 1 1 1 1
  spline S170 degree 3 poles (-29.3116, -18.6817) (-27.8828, -25.8921) (-23.5966, -32.0929) (-18.6912, -34.055) knots 0 0 0 0 1 1 1 1
  spline S171 degree 3 poles (-18.6912, -34.055) (-17.4053, -34.5694) (-16.4338, -34.7503) (-15.0526, -34.7503) knots 0 0 0 0 1 1 1 1
  spline S172 degree 3 poles (-15.0526, -34.7503) (-13.6048, -34.7408) (-12.9667, -34.5979) (-13.9668, -34.5027) knots 0 0 0 0 1 1 1 1
  spline S173 degree 3 poles (-13.9668, -34.5027) (-16.9957, -34.2169) (-20.339, -31.9214) (-22.8631, -28.3876) knots 0 0 0 0 1 1 1 1
  spline S174 degree 3 poles (-22.8631, -28.3876) (-23.587, -27.3685) (-25.1015, -24.7396) (-25.1015, -24.4824) knots 0 0 0 0 1 1 1 1
  spline S175 degree 3 poles (-25.1015, -24.4824) (-25.1015, -24.4443) (-24.8253, -24.8253) (-24.4824, -25.3396) knots 0 0 0 0 1 1 1 1
  spline S176 degree 3 poles (-24.4824, -25.3396) (-22.1678, -28.7972) (-18.7864, -31.75) (-15.1479, -33.493) knots 0 0 0 0 1 1 1 1
  spline S177 degree 3 poles (-15.1479, -33.493) (-12.2332, -34.8837) (-9.5186, -35.4838) (-6.623, -35.3504) knots 0 0 0 0 1 1 1 1
  spline S178 degree 3 poles (-6.623, -35.3504) (-4.4704, -35.2647) (-2.7749, -34.8361) (-1.0699, -33.9693) knots 0 0 0 0 1 1 1 1
  spline S179 degree 3 poles (-1.0699, -33.9693) (-0.2413, -33.5407) (1.4256, -32.4548) (1.3494, -32.3786) knots 0 0 0 0 1 1 1 1
  spline S180 degree 3 poles (1.3494, -32.3786) (1.3304, -32.3596) (0.997, -32.4548) (0.5969, -32.5786) knots 0 0 0 0 1 1 1 1
  spline S181 degree 3 poles (0.5969, -32.5786) (-1.0604, -33.1025) (-1.9653, -33.2359) (-4.0036, -33.2359) knots 0 0 0 0 1 1 1 1
  spline S182 degree 3 poles (-4.0036, -33.2359) (-6.3468, -33.2454) (-7.5374, -33.0549) (-9.8139, -32.3215) knots 0 0 0 0 1 1 1 1
  line L33 (-9.8139, -32.3215) -> (-10.7664, -32.0071)
  line L34 (-10.7664, -32.0071) -> (-9.5281, -31.95)
  spline S183 degree 3 poles (-9.5281, -31.95) (-8.2899, -31.8928) (-7.5374, -31.75) (-6.4992, -31.369) knots 0 0 0 0 1 1 1 1
  spline S184 degree 3 poles (-6.4992, -31.369) (-6.2039, -31.2642) (-5.9563, -31.1689) (-5.9563, -31.1594) knots 0 0 0 0 1 1 1 1
  spline S185 degree 3 poles (-5.9563, -31.1594) (-5.9563, -31.1499) (-6.5087, -31.1594) (-7.1945, -31.1785) knots 0 0 0 0 1 1 1 1
  spline S186 degree 3 poles (-7.1945, -31.1785) (-8.6995, -31.2261) (-9.671, -31.0927) (-10.995, -30.6641) knots 0 0 0 0 1 1 1 1
  spline S187 degree 3 poles (-10.995, -30.6641) (-16.6719, -28.8067) (-21.9392, -22.8441) (-24.53, -15.3384) knots 0 0 0 0 1 1 1 1
  spline S188 degree 3 poles (-24.53, -15.3384) (-24.9682, -14.062) (-25.4158, -12.4618) (-25.3682, -12.338) knots 0 0 0 0 1 1 1 1
  spline S189 degree 3 poles (-25.3682, -12.338) (-25.3492, -12.2904) (-25.0348, -12.4428) (-24.6729, -12.6809) knots 0 0 0 0 1 1 1 1
  spline S190 degree 3 poles (-24.6729, -12.6809) (-23.6347, -13.3572) (-21.0724, -14.5764) (-19.8056, -14.9955) knots 0 0 0 0 1 1 1 1
  spline S191 degree 3 poles (-19.8056, -14.9955) (-17.8054, -15.6622) (-16.9195, -15.8051) (-14.9098, -15.8146) knots 0 0 0 0 1 1 1 1
  spline S192 degree 3 poles (-14.9098, -15.8146) (-13.3572, -15.8146) (-13.0619, -15.7861) (-12.4047, -15.5956) knots 0 0 0 0 1 1 1 1
  spline S193 degree 3 poles (-12.4047, -15.5956) (-11.2141, -15.2527) (-10.4616, -14.8431) (-9.7663, -14.1478) knots 0 0 0 0 1 1 1 1
  spline S194 degree 3 poles (-9.7663, -14.1478) (-8.6899, -13.081) (-8.2708, -11.9189) (-8.3756, -10.2425) knots 0 0 0 0 1 1 1 1
  spline S195 degree 3 poles (-8.3756, -10.2425) (-8.4042, -9.6901) (-8.4518, -9.1376) (-8.4899, -9.0043) knots 0 0 0 0 1 1 1 1
  spline S196 degree 3 poles (-8.4899, -9.0043) (-8.5375, -8.7661) (-8.4994, -8.7376) (-7.4326, -8.3375) knots 0 0 0 0 1 1 1 1
  spline S197 degree 3 poles (-7.4326, -8.3375) (-6.4897, -7.9756) (-6.3182, -7.8803) (-6.2801, -7.6708) knots 0 0 0 0 1 1 1 1
  spline S198 degree 3 poles (-6.2801, -7.6708) (-4.918, -1.2795) (-0.1555, 3.4735) (5.6738, 4.2545) knots 0 0 0 0 1 1 1 1
  line L35 (5.6738, 4.2545) -> (6.5025, 4.3593)
  line L36 (6.5025, 4.3593) -> (6.5596, 4.7879)
  spline S199 degree 3 poles (6.5596, 4.7879) (6.6549, 5.4737) (6.6072, 6.912) (6.4834, 7.4454) knots 0 0 0 0 1 1 1 1
  spline S200 degree 3 poles (-10.814, -9.652) (-19.3294, -12.8714) (-27.1303, -12.3094) (-30.1879, -8.2423) knots 0 0 0 0 1 1 1 1
  spline S201 degree 3 poles (-30.1879, -8.2423) (-30.4355, -7.9089) (-30.6165, -7.6231) (-30.5879, -7.6041) knots 0 0 0 0 1 1 1 1
  spline S202 degree 3 poles (-30.5879, -7.6041) (-30.5689, -7.585) (-30.2736, -7.7851) (-29.9402, -8.0518) knots 0 0 0 0 1 1 1 1
  spline S203 degree 3 poles (-29.9402, -8.0518) (-29.2258, -8.6328) (-27.5685, -9.4614) (-26.3874, -9.852) knots 0 0 0 0 1 1 1 1
  spline S204 degree 3 poles (-26.3874, -9.852) (-22.625, -11.0617) (-17.7101, -11.0998) (-12.6619, -9.9472) knots 0 0 0 0 1 1 1 1
  spline S205 degree 3 poles (-12.6619, -9.9472) (-11.9856, -9.7948) (-11.0807, -9.5662) (-10.6616, -9.4329) knots 0 0 0 0 1 1 1 1
  spline S206 degree 3 poles (-10.6616, -9.4329) (-9.9377, -9.2043) (-9.6901, -9.1471) (-9.7758, -9.2329) knots 0 0 0 0 1 1 1 1
  spline S207 degree 3 poles (-9.7758, -9.2329) (-9.7948, -9.2519) (-10.2616, -9.4424) (-10.814, -9.652) knots 0 0 0 0 1 1 1 1
  point P0 (42.2474, 35.4497)
  point P1 (42.2474, -35.4497)
  point P2 (-42.2474, -35.4497)
  point P3 (-42.2474, 35.4497)
  point P4 (-42.2473, -35.4497)
  point P5 (-42.2474, 35.4497)
  point P6 (42.2443, -35.4374)
  point P7 (42.246, 35.4576)
  point P8 (-9.4894, 28.0017)
  point P9 (5.5003, 28.0002)
  point P10 (-9.5, -28)
  point P11 (5.5279, -27.9998)
  point P12 (-46.9939, 12.0456)
  dimension "d325" = 3
  dimension "d330" = 4
  dimension "d381" = 2.85
  dimension "d382" = 2.85
  dimension "d386" = 6
  dimension "d387" = 2.85
  dimension "d388" = 2.85
  dimension "d791" = 7
  dimension "d794" = 7
  dimension "d795" = 7
  dimension "d797" = 7
  dimension "d800" = 7
  dimension "d801" = 7
  dimension "d812" = 0.6
  dimension "d887" = 1
  dimension "d888" = 1
  dimension "d968" = 3
  dimension "d969" = 3
  dimension "d970" = 3
  dimension "d971" = 3
  dimension "d974" = 9
  dimension "d975" = 9
  dimension "d976" = 9
  dimension "d977" = 9
  dimension "d980" = 6.1
  dimension "d981" = 6.1
  dimension "d1003" = 5
  constraint horizontal L0
  constraint tangent A3 A12
  constraint tangent A2 A4
  constraint equal A3 A4
  constraint tangent A0 A5
  constraint tangent A0 A6
  constraint equal A5 A6
  constraint concentric A6 A7
  constraint concentric A5 A8
  constraint concentric A10 A14
  constraint concentric A11 A15
  constraint horizontal L1
  constraint coincident P5 P3
  constraint coincident P6 A2.centre
  constraint coincident P7 A12.centre
  constraint coincident A1 S0.end
  constraint midpoint S0.start L4
  constraint midpoint S0.end L5
  constraint concentric A15 A22
  constraint tangent L6 A16
  constraint tangent A14 A16
  constraint tangent L6 A17
  constraint tangent A14 A18
  constraint tangent S1 A18
  constraint tangent S1 A19
  constraint tangent A15 A19
  constraint tangent A15 A20
  constraint tangent S2 A20
  constraint tangent S2 A21
  constraint tangent L7 A23
  constraint tangent A13 A26
  constraint tangent A25 A26
  constraint tangent A17 A27
  constraint tangent A25 A27
  constraint tangent A1 A28
  constraint tangent A24 A28
  constraint tangent A24 A29
  constraint tangent A21 A29
  constraint equal A28 A29
  constraint concentric A30 A31
  constraint tangent L0 A32
  constraint tangent A1 A32
  constraint tangent L0 A33
  constraint tangent A2 A33
  constraint tangent L8 A34
  constraint tangent A12 A34
  constraint tangent L8 A35
  constraint tangent A13 A35
  constraint concentric A14 A36
  constraint concentric A22 A37
  constraint concentric A14 A38
  constraint concentric A37 A39
  constraint concentric A7 A41
  constraint coincident A30 A40.end
  constraint coincident A0 A40.start
  constraint coincident A0 A41.end
  constraint coincident A31 A41.start
  constraint concentric A40 A43
  constraint concentric A6 A42
  constraint coincident A31 A42.end
  constraint coincident A31 A42.start
  constraint coincident A30 A43.end
  constraint coincident A30 A43.start
  constraint coincident A39 A20.end
  constraint coincident A39 A19.start
  constraint coincident A38 A18.end
  constraint coincident A38 A16.start
  measures "d325" radius of A3
  measures "d330" radius of A5
  measures "d381" diameter of A7
  measures "d382" diameter of A8
  measures "d386" diameter of A15
  measures "d387" diameter of A10
  measures "d388" diameter of A11
  measures "d791" radius of A16
  measures "d794" radius of A17
  measures "d795" radius of A18
  measures "d797" radius of A19
  measures "d800" radius of A20
  measures "d801" radius of A21
  measures "d812" radius of A23
  measures "d887" radius of A27
  measures "d888" radius of A28
  measures "d968" radius of A32
  measures "d969" radius of A33
  measures "d970" radius of A34
  measures "d971" radius of A35
  measures "d974" diameter of A38
  measures "d975" diameter of A39
  measures "d976" diameter of A40
  measures "d977" diameter of A41
  measures "d980" diameter of A43
  measures "d981" diameter of A42
  measures "d1003" diameter of A44
extrude "Extrude155" add sketch "Sketch6" along normal blind 2.5 contours L0 A0 A1 A2 A9 A12 A13 L8 A32 A33 A34 A35 A38 A39 A40 A41 | A2 A4 A9 A30 A40 | A1 A9 S2 A20 A21 A24 A28 A29 A39 | A9 S1 A18 A19 A38 A39 | A3 A9 A12 A31 A41 | A9 A13 L6 A16 A17 A25 A26 A27 A38 | S99 S100 S101 S102 S103 | S200 S201 S202 S203 S204 S205 S206 S207 makes body 1 at (-4.4689, 0, -35.0341) makes body 2 at (21.9794, 0, 5.0539) makes body 3 at (-12.3905, 0.8333, 10.2078)
extrude "Extrude154" add sketch "Sketch6" along normal blind 4 contours A0 A5 A9 A40 A43 | A9 A30 A40 A43 | A9 A15 A37 A39 | A9 A37 A39 | A5 A9 A30 A43 | A0 A6 A9 A41 A42 | A9 A31 A41 A42 | A9 A14 A36 A38 | A9 A36 A38 | A6 A9 A31 A42 makes body 4 at (-50.3813, 1.3333, 12.405) makes body 5 at (57.7126, 2.6667, -21.0597) makes body 6 at (-50.3868, 1.3333, -12.1693) makes body 7 at (57.0413, 2.6667, 22.7991)
fillet "Fillet164" radius 0.5 2 edges at (-57.6727, 4, 11.0959) (-57.6782, 4, -13.4784) on bodies 4 6
fillet "Fillet174" radius 1 2 edges at (-59.0712, 4, 13.808) (-59.0767, 4, -10.7663) on bodies 4 6
extrude "Extrude156" add sketch "Sketch6" along normal blind 1.75 contours S3 S4 L9 L10 S5 S6 S7 S8 S9 S10 S11 S12 S13 S14 L11 L12 S15 S16 S17 L13 L14 S18 S19 S20 S21 S22 S23 S24 S25 S26 S27 S28 S29 S30 S31 L15 L16 S32 S33 S34 S35 L17 L18 S36 S37 S38 S39 S40 S41 S42 S43 S44 S45 S46 S47 S48 S49 S50 S51 S52 L19 L20 S53 S54 S55 S56 S57 S58 S59 S60 S61 S62 S63 S64 S65 S66 S67 S68 L21 L22 S69 S70 S71 S72 S73 S74 S75 S76 S77 S78 S79 S80 S81 S82 S83 S84 S85 S86 S87 S88 S89 L23 L24 S90 S91 S92 S93 S94 S95 S96 S97 S98 | S116 S117 S118 | S119 S120 S121 S122 S123 S124 S125 S126 S127 S128 S129 S130 S131 S132 S133 S134 S135 S136 S137 S138 S139 S140 S141 S142 L27 L28 S143 S144 S145 L29 L30 S146 S147 S148 S149 S150 S151 S152 S153 S154 S155 S156 L31 L32 S157 S158 S159 S160 S161 S162 S163 S164 S165 S166 S167 S168 S169 S170 S171 S172 S173 S174 S175 S176 S177 S178 S179 S180 S181 S182 L33 L34 S183 S184 S185 S186 S187 S188 S189 S190 S191 S192 S193 S194 S195 S196 S197 S198 L35 L36 S199 bodies 1 2 3
extrude "Extrude157" add sketch "Sketch6" along normal blind 2.5 contours A9 A43 | A9 A30 A43 | A9 A31 A42 | A9 A42 | A9 A10 A14 A36 | A9 A10 A36 | S104 S105 S106 S107 S108 S109 L25 L26 S110 S111 S112 S113 S114 S115 bodies 1 5 6 7
extrude "Extrude158" add sketch "Sketch6" along normal blind 2.5 contours A9 A11 A15 A37 | A9 A11 A37 bodies 4
combine "Combine5" operation add target body 1 tool bodies 5 6 4 7
fillet "Fillet176" radius 0.5 28 edges at (-54.9645, 2.5, 17.1097) (-54.562, 2.5, 18.3031) (-54.053, 2.5, 22.4021) (-55.5805, 2.5, 25.9917) (-55.2379, 2.5, 27.0408) (-54.1637, 2.5, 28.1039) (-37.1724, 2.5, 22.9406) (-28.2097, 2.5, 39.9541) (0.0083, 2.5, 41.0033) (28.2275, 2.5, 39.9527) (36.3501, 2.5, 23.2945) (53.5547, 2.5, 27.1153) (53.5254, 2.5, -27.1878) (36.389, 2.5, -23.3591) (28.2819, 2.5, -39.9518) (0.0346, 2.5, -41.0009) (-28.2118, 2.5, -39.9515) (-37.1797, 2.5, -22.9339) (-54.1805, 2.5, -28.0881) (-55.2543, 2.5, -27.0237) (-55.5967, 2.5, -25.9738) (-54.0676, 2.5, -22.38) (-54.5422, 2.5, -18.3977) (-54.9176, 2.5, -17.3227) (-57.4602, 2.5, -8.1942) (-58.517, 2.5, -0.0574) (-57.4836, 2.5, 8.0404) (29.5959, 2.5, 0.033) on bodies 1
